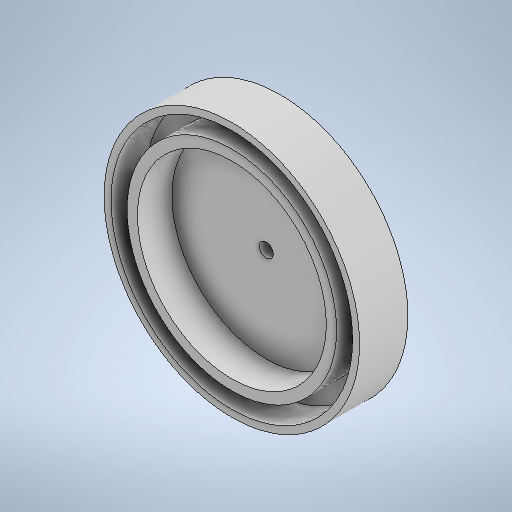
# Autodesk Inventor part: base_estable_soporte
Saved by Autodesk Inventor 2025.3 (Build 293356000, 356)
## iProperties
Created: 2025-08-17
Part Number: base_estable_soporte
Material: Genérico
Document SubType Name: Modeling
Designer: Rodrigo
Density: 1 g/cm^3
Appearance: Valor por defecto
Author: Rodrigo
## iProperties of the stored document base_estable_soporte_3DPrint.ipt
Created: 2025-08-17
Part Number: base_estable_soporte_3DPrint
Material: Genérico
Document SubType Name: Modeling
Designer: Rodrigo
Density: 1 g/cm^3
Appearance: Valor por defecto
Author: Rodrigo
Autodesk Inventor part; units mm, degrees
ref_plane "YZ Plane" through (0, 0, 0) normal (1, 0, 0) x (0, 1, 0)
ref_plane "XZ Plane" through (0, 0, 0) normal (0, 1, 0) x (-1, 0, 0)
ref_plane "XY Plane" through (0, 0, 0) normal (0, 0, 1) x (1, 0, 0)
sketch "Boceto1" plane through (0, 0, 0) normal (0, 0, 1) x (1, 0, 0)
  circle A0 centre (0, 0) radius 30.35
  circle A1 centre (0, 0) radius 35
  circle A2 centre (0, 0) radius 27.35
  circle A3 centre (0, 0) radius 37
  dimension "d0" = 60.7
  dimension "d1" = 70
  dimension "d2" = 3
  dimension "d3" = 2
  constraints: 4 centre point, 2 coincident
  measures "d0" diameter of A0
  measures "d1" diameter of A1
  measures "d2" radial gap between concentric circles of A0 A2
  measures "d3" radial gap between concentric circles of A1 A3
extrude "Extrusión1" add sketch "Boceto1" along normal blind 10
sketch "Boceto2" plane through (0, 0, 0) normal (0, 0, -1) x (-1, 0, 0)
  circle A0 centre (0, 0) radius 30.35
  circle A1 centre (0, 0) radius 35
  circle A2 centre (0, 0) radius 37
  constraints: 3 centre point, 3 coincident
extrude "Extrusión2" add sketch "Boceto2" along normal blind 4 contours A0 | A1 | A2
sketch "Boceto3" plane through (0, 0, -4) normal (0, 0, -1) x (-1, 0, 0)
  circle A0 centre (0, 0) radius 2
  dimension "d8" = 4
  constraints: 1 centre point, 1 coincident
  measures "d8" diameter of A0
extrude "Extrusión3" cut sketch "Boceto3" against normal blind 4
